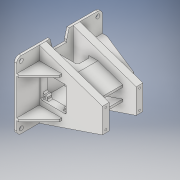
# Autodesk Inventor part: MotorSupport
Saved by Autodesk Inventor 2019.3 (Build 233278000, 278)
## iProperties
Created: 2019-06-25
Part Number: MotorSupport
Material: PC/ABS Plastic
Document SubType Name: Modeling
Designer: mark
Density: 0.357273 g/cm^3
Appearance: Smooth - White
Author: mark
Autodesk Inventor part; units mm, degrees
ref_plane "YZ Plane" through (0, 0, 0) normal (1, 0, 0) x (0, 1, 0)
ref_plane "XZ Plane" through (0, 0, 0) normal (0, 1, 0) x (-1, 0, 0)
ref_plane "XY Plane" through (0, 0, 0) normal (0, 0, 1) x (1, 0, 0)
sketch "Sketch1" plane through (0, 0, 0) normal (0, 0, 1) x (1, 0, 0)
  circle A0 centre (12.7, 19.05) radius 4 projected
  line L0 (-1.3, 46.55) -> (-1.3, -8.45)
  line L1 (-1.3, -8.45) -> (-141.3, -55.95)
  line L2 (-141.3, -55.95) -> (-141.3, 94.05)
  line L3 (-141.3, 94.05) -> (-1.3, 46.55)
  point P0 (0, 0)
  dimension "d0" = 55
  dimension "d1" = 27.5
  dimension "d2" = 14
  dimension "d3" = 150
  dimension "d4" = 140
  constraints: 8 end point, 2 vertical, 1 equal length
  measures "d0" distance of L0.end L0.start
  measures "d1" vertical distance of L0.start A0.centre
  measures "d2" distance from line of L0 A0.centre
  measures "d3" distance of L1.end L2.end
  measures "d4" distance between parallel lines of L2 L0
extrude "Extrusion1" add sketch "Sketch1" along normal blind 15 contours L0 L1 L2 L3
sketch "Sketch2" plane through (-141.3, -55.95, 0) normal (-1, 0, 0) x (0, 0, 1)
  line L0 (0, 0) -> (0, 150) projected
  line L1 (0, 0) -> (15, 0) projected
  line L2 (15, 150) -> (15, 0) projected
  line L3 (0, 150) -> (15, 150) projected
  point P0 (0, 55.95)
extrude "Extrusion2" add sketch "Sketch2" along normal blind 5
sketch "Sketch3" plane through (0, 0, 0) normal (0, 0, -1) x (-1, 0, 0)
  line L0 (1.3, 46.55) -> (1.3, -8.45) projected
  line L1 (1.3, -8.45) -> (141.3, -55.95) projected
  line L2 (141.3, -55.95) -> (146.3, -55.95) projected
  line L3 (146.3, 94.05) -> (146.3, -55.95) projected
  line L4 (141.3, 94.05) -> (146.3, 94.05) projected
  line L5 (141.3, 94.05) -> (1.3, 46.55) projected
  point P0 (0, 0)
extrude "Extrusion3" add sketch "Sketch3" along normal blind 75
sketch "Sketch4" plane through (-146.3, -55.95, 15) normal (0, -1, 0) x (1, 0, 0)
  line L0 (145, 0) -> (145, -90) projected
  line L1 (5, 0) -> (145, 0) projected
  line L2 (5, 0) -> (5, -90) projected
  line L3 (145, -90) -> (5, -90) projected
  line L4 (5, -15) -> (145, -15)
  line L5 (145, -15) -> (145, -75)
  line L6 (145, -75) -> (5, -75)
  line L7 (5, -75) -> (5, -15)
  point P0 (146.3, -15)
  dimension "d11" = 15
  dimension "d12" = 15
  constraints: 8 end point, 2 collinear
  measures "d11" distance between parallel lines of L1 L4
  measures "d12" distance between parallel lines of L3 L6
extrude "Extrusion4" cut sketch "Sketch4" against normal up to surface (150 mm away) contours L0 L6 L2 L4
sketch "Sketch5" plane through (-146.3, -55.95, 15) normal (0, -1, 0) x (1, 0, 0)
  line L0 (5, -29.125) -> (0, -29.125)
  line L1 (0, -29.125) -> (0, -60.875)
  line L2 (0, -60.875) -> (5, -60.875)
  line L3 (5, -60.875) -> (5, -29.125)
  line L4 (5, -15) -> (5, -75) projected
  line L5 (0, 0) -> (0, -90) projected
  line L6 (5, -90) -> (0, -90) projected
  point P0 (146.3, -15)
  dimension "d15" = 31.75
  dimension "d16" = 29.125
  constraints: 8 end point, 2 collinear, 1 horizontal
  measures "d15" distance of L2.end L0.start
  measures "d16" distance between parallel lines of L6 L2
extrude "Extrusion5" cut sketch "Sketch5" against normal blind 25
sketch "Sketch6" plane through (0, 0, 15) normal (0, 0, 1) x (1, 0, 0)
  line L0 (-1.3, -8.45) -> (-1.3, 46.55) projected
  line L1 (-1.3, 46.55) -> (-141.3, 94.05) projected
  line L2 (-141.3, 94.05) -> (-146.3, 94.05) projected
  line L3 (-146.3, -55.95) -> (-146.3, 94.05) projected
  line L4 (-141.3, -55.95) -> (-146.3, -55.95) projected
  line L5 (-141.3, -55.95) -> (-1.3, -8.45) projected
  line L6 (-141.3, 94.05) -> (-1.3, 46.55) projected
  line L7 (-141.3, 94.05) -> (-141.3, -55.95)
  line L8 (-141.3, 94.05) -> (-146.3, 94.05)
  line L9 (-146.3, -55.95) -> (-146.3, 94.05) projected
  line L10 (-141.3, -55.95) -> (-146.3, -55.95) projected
  line L11 (-146.3, -55.95) -> (-141.3, -55.95)
  point P0 (0, 0)
  constraints: 6 end point
extrude "Extrusion6" add sketch "Sketch6" along normal blind 50 contours L4 L3 L2 L7
sketch "Sketch7" plane through (0, 0, -75) normal (0, 0, -1) x (-1, 0, 0)
  line L0 (146.3, -55.95) -> (146.3, -30.95) projected
  line L1 (146.3, 94.05) -> (141.3, 94.05) projected
  line L2 (146.3, -55.95) -> (141.3, -55.95)
  line L3 (141.3, -55.95) -> (141.3, 94.05)
  line L4 (141.3, 94.05) -> (146.3, 94.05)
  line L5 (146.3, 94.05) -> (146.3, -55.95)
  point P0 (0, 0)
  constraints: 8 end point, 2 vertical
extrude "Extrusion7" add sketch "Sketch7" along normal blind 50
sketch "Sketch8" plane through (-141.3, -55.95, -60) normal (1, 0, 0) x (0, 0, -1)
  circle A0 centre (-115, 140) radius 4.5
  circle A1 centre (-115, 10) radius 4.5
  circle A2 centre (55, 10) radius 4.5
  circle A3 centre (55, 140) radius 4.5
  line L0 (-125, 0) -> (-125, 150) projected
  line L1 (-75, 150) -> (-125, 150) projected
  line L2 (-75, 0) -> (-125, 0) projected
  line L3 (65, 150) -> (65, 0) projected
  line L4 (15, 150) -> (65, 150) projected
  line L5 (15, 0) -> (65, 0) projected
  point P0 (-60, 55.95)
  dimension "d23" = 9
  dimension "d24" = 9
  dimension "d25" = 9
  dimension "d26" = 9
  dimension "d27" = 10
  dimension "d28" = 10
  dimension "d29" = 10
  dimension "d30" = 10
  dimension "d31" = 10
  dimension "d32" = 10
  dimension "d33" = 10
  dimension "d34" = 10
  constraints: 4 centre point
  measures "d23" diameter of A0
  measures "d24" diameter of A1
  measures "d25" diameter of A2
  measures "d26" diameter of A3
  measures "d27" distance from line of L0 A0.centre
  measures "d28" distance from line of L1 A0.centre
  measures "d29" distance from line of L2 A1.centre
  measures "d30" distance from line of L0 A1.centre
  measures "d31" distance from line of L3 A3.centre
  measures "d32" distance from line of L4 A3.centre
  measures "d33" distance from line of L3 A2.centre
  measures "d34" distance from line of L5 A2.centre
extrude "Extrusion8" cut sketch "Sketch8" against normal up to next
sketch "Sketch9" plane through (-141.3, -55.95, -60) normal (1, 0, 0) x (0, 0, -1)
  line L0 (15, 102.5) -> (65, 102.5)
  line L1 (65, 102.5) -> (65, 97.5)
  line L2 (65, 97.5) -> (15, 97.5)
  line L3 (15, 97.5) -> (15, 102.5)
  line L4 (15, 52.5) -> (65, 52.5)
  line L5 (65, 52.5) -> (65, 47.5)
  line L6 (65, 47.5) -> (15, 47.5)
  line L7 (15, 47.5) -> (15, 52.5)
  line L8 (15, 150) -> (15, 102.5) projected
  line L9 (15, 102.5) -> (15, 47.5) projected
  line L10 (65, 150) -> (65, 0) projected
  line L11 (15, 150) -> (65, 150) projected
  line L12 (15, 102.5) -> (0, 102.5) projected
  line L13 (0, 47.5) -> (15, 47.5) projected
  point P0 (40, 97.5)
  dimension "d77" = 5
  constraints: 16 end point, 7 collinear, 4 horizontal, 1 midpoint
  measures "d77" distance of L0.end L1.end
extrude "Extrusion9" add sketch "Sketch9" along normal blind 110 contours L0 L1 L2 L3 | L4 L5 L6 L7
chamfer "Chamfer3" distance 40 distance2 100 1 edges at (-31.3, -5.95, -125) measured on face at (-31.3, -5.1167, -91.6667)
chamfer "Chamfer4" distance 40 distance2 100 1 edges at (-31.3, 44.05, -125) measured on face at (-31.3, 44.8833, -91.6667)
fillet "Fillet1" radius 10 4 edges at (-143.8, 94.05, 65) (-143.8, -55.95, 65) (-143.8, -55.95, -125) (-143.8, 94.05, -125)
chamfer "Chamfer5" distance 20 angle 15 1 edges at (-143.8, -55.95, -45.875) measured on face at (-144.6333, -47.6167, -45.875)
chamfer "Chamfer6" distance 20 angle 15 1 edges at (-143.8, -55.95, -14.125) measured on face at (-142.9667, -47.6167, -14.125)
sketch "Sketch10" plane through (-1.3, -8.45, 15) normal (1, 0, 0) x (0, 0, -1)
  circle A0 centre (7.5, 48.75) radius 2
  circle A1 centre (7.5, 6.25) radius 2
  circle A2 centre (82.5, 6.25) radius 2
  circle A3 centre (82.5, 48.75) radius 2
  line L0 (15, 0) -> (15, 55) projected
  line L1 (90, 55) -> (90, 0) projected
  line L2 (0, 0) -> (0, 55) projected
  line L3 (90, 55) -> (75, 55) projected
  line L4 (15, 55) -> (0, 55) projected
  point P0 (15, 8.45)
  dimension "d61" = 7.5
  dimension "d62" = 7.5
  dimension "d63" = 7.5
  dimension "d64" = 7.5
  dimension "d65" = 42.5
  dimension "d66" = 42.5
  dimension "d67" = 6.25
  dimension "d68" = 6.25
  dimension "d69" = 4
  dimension "d70" = 4
  dimension "d71" = 4
  dimension "d72" = 4
  constraints: 4 centre point
  measures "d61" distance from line of L0 A0.centre
  measures "d62" distance from line of L1 A3.centre
  measures "d63" distance from line of L1 A2.centre
  measures "d64" distance from line of L2 A1.centre
  measures "d65" distance of A1.centre A0.centre
  measures "d66" distance of A2.centre A3.centre
  measures "d67" distance from line of A3.centre L3
  measures "d68" distance from line of L4 A0.centre
  measures "d69" diameter of A0
  measures "d70" diameter of A1
  measures "d71" diameter of A3
  measures "d72" diameter of A2
extrude "Extrusion10" cut sketch "Sketch10" against normal blind 25
sketch "Sketch11" plane through (0, 0, 15) normal (0, 0, 1) x (1, 0, 0)
  circle A0 centre (-111.3, 19.05) radius 19.05
  line L0 (-141.3, 94.05) -> (-141.3, -55.95) projected
  line L1 (-1.3, 46.55) -> (-141.3, 94.05) projected
  line L2 (-1.3, 46.55) -> (-1.3, -8.45) projected
  point P0 (0, 0)
  point P1 (-133.8764, 44.9804)
  point P2 (-135.7236, 40.1196)
  point P3 (-133.8764, -2.0196)
  point P4 (-135.7236, -6.8804)
  point P5 (-86.8764, -2.0196)
  point P6 (-88.7236, -6.8804)
  point P7 (-82.4146, 74.071)
  dimension "d82" = 38.1
  dimension "d153" = 27.5
  dimension "d154" = 110
  constraints: 1 centre point, 1 point on line
  measures "d82" diameter of A0
  measures "d153" vertical distance of A0.centre L1.start
  measures "d154" distance from line of L2 A0.centre
extrude "Extrusion11" cut sketch "Sketch11" against normal up to next
sketch "Sketch12" plane through (-141.3, 94.05, 0) normal (0, 1, 0) x (1, 0, 0)
  line L0 (0, 45.875) -> (-5, 45.875)
  line L1 (-5, 45.875) -> (-5, 14.125)
  line L2 (-5, 14.125) -> (0, 14.125)
  line L3 (0, 14.125) -> (0, 45.875)
  line L4 (0, -15) -> (0, -75)
  line L5 (-5, 0) -> (-5, -15)
  line L6 (5, -15) -> (-5, -15)
  line L7 (-5, 115) -> (-5, -55) projected
  line L8 (0, 60) -> (0, 0) projected
  line L9 (140, -15) -> (0, -15) projected
  point P0 (141.3, 0)
  point P1 (131.3, -15)
  point P2 (39.1779, -15)
  dimension "d110" = 31.75
  dimension "d111" = 29.125
  constraints: 14 end point, 5 collinear, 1 horizontal
  measures "d110" distance of L2.end L0.start
  measures "d111" distance between parallel lines of L6 L2
extrude "Extrusion12" cut sketch "Sketch12" against normal blind 25
chamfer "Chamfer7" distance 20 angle 15 1 edges at (-143.8, 94.05, -45.875) measured on face at (-142.9667, 85.7167, -45.875)
chamfer "Chamfer8" distance 20 angle 15 1 edges at (-143.8, 94.05, -14.125) measured on face at (-144.6333, 85.7167, -14.125)
sketch "Sketch13" plane through (-141.3, -55.95, 0) normal (1, 0, 0) x (0, 0, -1)
  line L0 (60, 40) -> (0, 40)
  line L1 (0, 40) -> (0, 45)
  line L2 (0, 45) -> (60, 45)
  line L3 (60, 45) -> (60, 40)
  line L4 (60, 47.5) -> (60, 0) projected
  line L5 (0, 0) -> (0, 47.5) projected
  line L6 (0, 79.3248) -> (0, 74.2943) projected
  line L7 (14.125, 25) -> (45.875, 25) projected
  line L8 (60, 110) -> (0, 110)
  line L9 (0, 110) -> (0, 105)
  line L10 (0, 105) -> (60, 105)
  line L11 (60, 105) -> (60, 110)
  line L12 (45.875, 125) -> (14.125, 125) projected
  point P0 (0, 55.95)
  point P1 (0, 74.4639)
  dimension "d120" = 5
  dimension "d184" = 15
  dimension "d185" = 5
  dimension "d186" = 15
  constraints: 16 end point, 4 collinear, 1 horizontal
  measures "d120" distance between parallel lines of L2 L0
  measures "d184" distance between parallel lines of L0 L7
  measures "d185" distance between parallel lines of L10 L8
  measures "d186" distance between parallel lines of L12 L8
extrude "MidRibs" add sketch "Sketch13" along normal blind 55
sketch "Sketch17" plane through (-141.3, -55.95, 15) normal (1, 0, 0) x (0, 0, -1)
  line L0 (0, 30) -> (-50, 30)
  line L1 (-50, 30) -> (-50, 35)
  line L2 (-50, 35) -> (0, 35)
  line L3 (0, 35) -> (0, 30)
  line L4 (-50, 10) -> (-50, 140) projected
  line L5 (0, 0) -> (0, 47.5) projected
  line L6 (140, 97.5) -> (140, 102.5) projected
  line L7 (0, 0) -> (-40, 0) projected
  line L8 (-50, 120) -> (0, 120)
  line L9 (0, 120) -> (0, 115)
  line L10 (0, 115) -> (-50, 115)
  line L11 (-50, 115) -> (-50, 120)
  line L12 (0, 150) -> (-40, 150) projected
  line L13 (0, 102.5) -> (0, 150) projected
  point P0 (15, 55.95)
  dimension "d142" = 30
  dimension "d187" = 30
  constraints: 16 end point, 4 collinear, 2 equal length, 1 horizontal, 1 parallel
  measures "d142" distance between parallel lines of L0 L7
  measures "d187" distance between parallel lines of L12 L8
extrude "MotorFaceRib" add sketch "Sketch17" along normal blind 50
chamfer "Chamfer9" distance 45 angle 45 2 edges at (-91.3, -23.45, 65) (-91.3, 61.55, 65)
sketch "Sketch18" plane through (0, 0, 15) normal (0, 0, 1) x (1, 0, 0)
  line L0 (-137.8, -6.2) -> (-137.8, 44.3)
  line L1 (-134.8, 47.3) -> (-84.3, 47.3)
  line L2 (-81.3, 44.3) -> (-81.3, -6.2)
  line L3 (-84.3, -9.2) -> (-134.8, -9.2)
  circle A0 centre (-111.3, 19.05) radius 19.05 projected
  arc A1 (-134.8, 47.3) -> (-137.8, 44.3) centre (-134.8, 44.3) ccw
  arc A2 (-81.3, 44.3) -> (-84.3, 47.3) centre (-84.3, 44.3) ccw
  arc A3 (-84.3, -9.2) -> (-81.3, -6.2) centre (-84.3, -6.2) ccw
  arc A4 (-137.8, -6.2) -> (-134.8, -9.2) centre (-134.8, -6.2) ccw
  point P0 (0, 0)
  dimension "d157" = 56.5
  dimension "d158" = 56.5
  dimension "d159" = 28.25
  dimension "d160" = 30
  dimension "d161" = 3
  constraints: 8 end point, 8 point on circle, 8 tangent, 4 centre point, 3 equal radius, 1 horizontal, 1 vertical
  measures "d157" distance between parallel lines of L1 L3
  measures "d158" distance between parallel lines of L2 L0
  measures "d159" distance from line of L1 A0.centre
  measures "d160" distance from line of L2 A0.centre
  measures "d161" radius of A1
extrude "MotorIndent" cut sketch "Sketch18" against normal blind 5
sketch "Sketch19" plane through (0, 0, 10) normal (0, 0, 1) x (1, 0, 0)
  circle A0 centre (-133.3, 42.55) radius 2
  circle A1 centre (-86.3, 42.55) radius 2
  circle A2 centre (-86.3, -4.45) radius 2
  circle A3 centre (-133.3, -4.45) radius 2
  line L0 (-128.55, 41.05) -> (-128.55, 44.3)
  line L1 (-134.8, 47.3) -> (-84.3, 47.3) projected
  line L2 (-90.55, 44.3) -> (-90.55, 41.05)
  line L3 (-87.55, 38.05) -> (-84.3, 38.05)
  line L4 (-84.3, 0.05) -> (-87.55, 0.05)
  line L5 (-90.55, -2.95) -> (-90.55, -6.2)
  line L6 (-128.55, -6.2) -> (-128.55, -2.95)
  line L7 (-141.3, 41.55) -> (-141.3, -3.45) projected
  circle A4 centre (-111.3, 19.05) radius 19.05 projected
  line L8 (-141.3, -20.95) -> (-141.3, 84.05) projected
  line L9 (-81.3, 44.3) -> (-81.3, -6.2) projected
  line L10 (-84.3, -9.2) -> (-134.8, -9.2) projected
  line L11 (-137.8, -6.2) -> (-137.8, 44.3) projected
  line L12 (-131.55, 38.05) -> (-134.8, 38.05)
  line L13 (-131.55, 0.05) -> (-134.8, 0.05)
  arc A5 (-131.55, 38.05) -> (-128.55, 41.05) centre (-131.55, 41.05) ccw
  arc A6 (-90.55, 41.05) -> (-87.55, 38.05) centre (-87.55, 41.05) ccw
  arc A7 (-87.55, 0.05) -> (-90.55, -2.95) centre (-87.55, -2.95) ccw
  arc A8 (-128.55, -2.95) -> (-131.55, 0.05) centre (-131.55, -2.95) ccw
  line L14 (-125.55, 47.3) -> (-93.55, 47.3)
  line L15 (-81.3, 35.05) -> (-81.3, 3.05)
  line L16 (-93.55, -9.2) -> (-125.55, -9.2)
  line L17 (-137.8, 3.05) -> (-137.8, 35.05)
  arc A9 (-125.55, 47.3) -> (-128.55, 44.3) centre (-125.55, 44.3) ccw
  arc A10 (-90.55, 44.3) -> (-93.55, 47.3) centre (-93.55, 44.3) ccw
  arc A11 (-81.3, 35.05) -> (-84.3, 38.05) centre (-84.3, 35.05) ccw
  arc A12 (-84.3, 0.05) -> (-81.3, 3.05) centre (-84.3, 3.05) ccw
  arc A13 (-93.55, -9.2) -> (-90.55, -6.2) centre (-93.55, -6.2) ccw
  arc A14 (-128.55, -6.2) -> (-125.55, -9.2) centre (-125.55, -6.2) ccw
  arc A15 (-137.8, 3.05) -> (-134.8, 0.05) centre (-134.8, 3.05) ccw
  arc A16 (-134.8, 38.05) -> (-137.8, 35.05) centre (-134.8, 35.05) ccw
  point P0 (0, 0)
  point P1 (-128.55, 47.3)
  point P2 (-90.55, 47.3)
  point P3 (-81.3, 38.05)
  point P4 (-81.3, 0.05)
  point P5 (-90.55, -9.2)
  point P6 (-128.55, -9.2)
  point P7 (-137.8, 38.05)
  point P8 (-137.8, 0.05)
  dimension "d164" = 4
  dimension "d165" = 47
  dimension "d166" = 23.5
  dimension "d167" = 47
  dimension "d168" = 47
  dimension "d169" = 47
  dimension "d173" = 23.5
  dimension "d176" = 4.5
  dimension "d177" = 4.5
  dimension "d178" = 9.25
  dimension "d179" = 9.25
  dimension "d180" = 3
  dimension "d181" = 3
  constraints: 24 end point, 24 point on circle, 24 point on line, 24 tangent, 16 centre point, 13 equal radius, 6 equal length, 4 horizontal, 3 vertical
  measures "d164" diameter of A0
  measures "d165" distance of A3.centre A0.centre
  measures "d166" vertical distance of A4.centre A0.centre
  measures "d167" distance of A1.centre A0.centre
  measures "d168" distance of A2.centre A1.centre
  measures "d169" distance of A3.centre A2.centre
  measures "d173" vertical distance of A1.centre A4.centre
  measures "d176" distance from line of L11 A0.centre
  measures "d177" distance from line of L11 A3.centre
  measures "d178" distance between parallel lines of L1 L12
  measures "d179" distance between parallel lines of L11 L0
  measures "d180" radius of A5
  measures "d181" radius of A9
extrude "MotorHole" cut sketch "Sketch19" against normal up to surface (10 mm away)
sketch "Sketch20" plane through (-1.3, -8.45, -60) normal (0, 0, 1) x (1, 0, 0)
  line L0 (-85, -2.5) -> (-85, -7.5) projected
  line L1 (-85, 62.5) -> (-85, 57.5) projected
  line L2 (-85, 57.5) -> (-30, 38.8393)
  line L3 (-30, 38.8393) -> (-30, 43.8393)
  line L4 (-30, 43.8393) -> (-85, 62.5)
  line L5 (-85, -2.5) -> (-30, 16.1607)
  line L6 (-30, 16.1607) -> (-30, 11.1607)
  line L7 (-30, 11.1607) -> (-85, -7.5)
  line L8 (0, 55) -> (0, 0) projected
  line L9 (-140, 102.5) -> (0, 55) projected
  line L10 (0, 0) -> (-140, -47.5) projected
  point P0 (1.3, 8.45)
  dimension "d189" = 30
  constraints: 12 end point, 5 parallel, 2 collinear
  measures "d189" distance between parallel lines of L8 L3
extrude "Extrusion19" add sketch "Sketch20" along normal up to next
sketch "Sketch21" plane through (-141.3, 54.05, 0) normal (0, 1, 0) x (1, 0, 0)
  line L0 (35, 60) -> (0, 60)
  line L1 (0, 60) -> (0, 30)
  line L2 (0, 30) -> (35, 30)
  line L3 (40, 35) -> (40, 55)
  line L4 (0, 45.875) -> (0, 14.125) projected
  line L5 (0, 60) -> (140, 60) projected
  line L6 (35, 60) -> (40, 55)
  line L7 (35, 30) -> (40, 35)
  point P0 (141.3, 0)
  point P1 (40, 60)
  point P2 (40, 30)
  dimension "d195" = 30
  dimension "d196" = 40
  dimension "d197" = 5
  dimension "d198" = 5
  dimension "d199" = 5
  dimension "d200" = 5
  constraints: 12 end point, 4 point on line, 2 collinear
  measures "d195" distance between parallel lines of L2 L0
  measures "d196" distance between parallel lines of L1 L3
  measures "d197" distance of L0.start point (40, 60)
  measures "d198" distance of L3.end point (40, 60)
  measures "d199" distance of L2.end point (40, 30)
  measures "d200" distance of L3.start point (40, 30)
extrude "Extrusion20" cut sketch "Sketch21" against normal up to next
body "Solid1"
